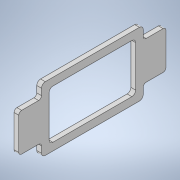
# Autodesk Inventor part: GRS104_hygrometer_fixture
Saved by Autodesk Inventor 2022.5 (Build 265521000, 521)
## iProperties
Created: 2024-01-17
Part Number: GRS104_hygrometer_fixture
Material: 一般
Document SubType Name: Modeling
Designer: gakut
Density: 1 g/cm^3
Appearance: 既定
Author: gakut
## iProperties of the stored document GRS104_hygrometer_fixture_3D プリント.ipt
Created: 2024-01-17
Part Number: GRS104_hygrometer_fixture_3D プリント
Material: 一般
Document SubType Name: Modeling
Designer: gakut
Density: 1 g/cm^3
Appearance: 既定
Author: gakut
Autodesk Inventor part; units mm, degrees
ref_plane "YZ Plane" through (0, 0, 0) normal (1, 0, 0) x (0, 1, 0)
ref_plane "XZ Plane" through (0, 0, 0) normal (0, 1, 0) x (-1, 0, 0)
ref_plane "XY Plane" through (0, 0, 0) normal (0, 0, 1) x (1, 0, 0)
sketch "スケッチ1" plane through (0, 0, 0) normal (1, 0, 0) x (0, 1, 0)
  line L0 (-12.85, 22.85) -> (12.85, 22.85)
  line L1 (12.85, 22.85) -> (12.85, -22.85)
  line L2 (12.85, -22.85) -> (-12.85, -22.85)
  line L3 (-12.85, -22.85) -> (-12.85, 22.85)
  line L4 (-12.85, 22.85) -> (12.85, -22.85) construction
  line L5 (12.85, 22.85) -> (-12.85, -22.85) construction
  line L6 (16.85, -26.85) -> (16.85, 26.85)
  line L7 (16.85, 26.85) -> (-16.85, 26.85)
  line L8 (-16.85, 26.85) -> (-16.85, -26.85)
  line L9 (-16.85, -26.85) -> (16.85, -26.85)
  line L10 (-10, 14.85) -> (10, 14.85)
  line L11 (10, 14.85) -> (10, 38.85)
  line L12 (10, 38.85) -> (-10, 38.85)
  line L13 (-10, 38.85) -> (-10, 14.85)
  line L14 (-10, 14.85) -> (10, 38.85) construction
  line L15 (10, 14.85) -> (-10, 38.85) construction
  line L16 (-10, -14.85) -> (10, -14.85)
  line L17 (10, -14.85) -> (10, -38.85)
  line L18 (10, -38.85) -> (-10, -38.85)
  line L19 (-10, -38.85) -> (-10, -14.85)
  line L20 (-10, -14.85) -> (10, -38.85) construction
  line L21 (10, -14.85) -> (-10, -38.85) construction
  point P0 (0, 0)
  point P1 (0, 26.85)
  point P2 (0, -26.85)
  point P3 (10, -26.85)
  point P4 (-10, -26.85)
  point P5 (-10, 26.85)
  point P6 (10, 26.85)
  dimension "d0" = 25.7
  dimension "d1" = 45.7
  dimension "d2" = 4
  dimension "d5" = 12
  dimension "d6" = 12
  dimension "d7" = 20
  dimension "d8" = 20
  constraints: 44 end point, 8 midpoint, 8 parallel, 4 perpendicular, 3 horizontal, 3 other
  measures "d0" distance of L1.end L2.end
  measures "d1" distance of L0.end L1.end
  measures "d2" distance between parallel lines of L1 L6
  measures "d5" distance between parallel lines of L7 L12
  measures "d6" distance between parallel lines of L18 L9
  measures "d7" distance of L11.end L12.end
  measures "d8" distance of L17.end L18.end
extrude "押し出し1" add sketch "スケッチ1" along normal blind 2.5 contours L3 L2 L19 L9 L8 L7 L13 L0 | L13 L7 L11 L0 | L11 L7 L6 L9 L17 L2 L1 L0 | L13 L12 L11 L7 | L2 L17 L9 L19 | L9 L17 L18 L19
fillet "フィレット1" radius 2 8 edges at (1.25, 12.85, 22.85) (1.25, 12.85, -22.85) (1.25, -12.85, -22.85) (1.25, -12.85, 22.85) (1.25, -16.85, 26.85) (1.25, 16.85, 26.85) (1.25, -16.85, -26.85) (1.25, 16.85, -26.85)
fillet "フィレット2" radius 1.5 8 edges at (1.25, 10, 26.85) (1.25, 10, 38.85) (1.25, -10, 38.85) (1.25, -10, 26.85) (1.25, -10, -26.85) (1.25, -10, -38.85) (1.25, 10, -26.85) (1.25, 10, -38.85)
equation "\"d6\" = d5"
equation "\"d8\" = d7"
